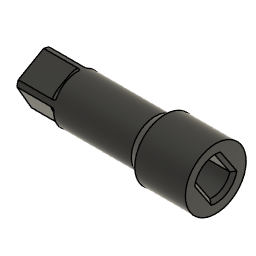
327ee1e9-15fe-45b5-88e0-88bf1f6365e6 (Autodesk Fusion 360 design; units mm, degrees)
Autodesk Fusion 360 part; units mm, degrees
sketch "Esboço1" plane through (-18.5, 0, 0) normal (-1, 0, 0) x (0, 0.065186, -0.997873)
  circle A0 centre (-39.8924, -6.2763) radius 4.5
  line L0 (-38.1174, -4.275) -> (-38.1174, -8.2775)
  line L1 (-41.6674, -4.275) -> (-41.6674, -8.2775)
  arc A1 (-41.6674, -8.2775) -> (-38.1174, -8.2775) centre (-39.8924, -6.2763) ccw
  arc A2 (-38.1174, -4.275) -> (-41.6674, -4.275) centre (-39.8924, -6.2763) ccw
  line L2 (-38.1174, -6.2763) -> (-41.6674, -6.2763) construction
  dimension "d5" = 9
  dimension "d16" = 5.35
  dimension "d18" = 3.55
  constraint vertical L1
  constraint coincident L0.start A1
  constraint concentric A1 A2
  constraint concentric A0 A2
  constraint coincident L0 L2.start
  constraint coincident L1 L2.end
  constraint perpendicular L1 L2
  constraint midpoint A0.centre L2
  constraint perpendicular L0 L2
  measures "d5" diameter of A0
  measures "d16" diameter of A1
  measures "d18" distance of L0 L1
extrude "Extrusão1" add sketch "Esboço1" against normal blind 7.5 contours A0 | L0 L1 A1 A2
sketch "Esboço2" plane through (-18.5, 0, 0) normal (-1, 0, 0) x (0, -1, 0)
  circle A0 centre (-3.6625, 40.2167) radius 4.5
  circle A1 centre (-3.6625, 40.2167) radius 3.5
  dimension "d9" = 7
  constraint concentric A0 A1
  measures "d9" diameter of A1
extrude "Extrusão3" cut sketch "Esboço1" against normal blind 7.5 contours L0 L1 A1 A2
extrude "Extrusão2" add sketch "Esboço2" along normal blind 13 contours A1
chamfer "Chanfro1" distance 1 distance2 1.5 1 edges at (-18.5, 6.9256, 41.4824) measured on face at (-18.5, 4.1672, 36.091)
sketch "Esboço3" plane through (-31.5, 0, 0) normal (-1, 0, 0) x (0, -1, 0)
  circle A0 centre (-3.6625, 40.2167) radius 3.5
  line L0 (-0.9125, 42.9667) -> (-6.4125, 42.9667)
  line L1 (-6.4125, 42.9667) -> (-6.4125, 37.4667)
  line L2 (-6.4125, 37.4667) -> (-0.9125, 37.4667)
  line L3 (-0.9125, 37.4667) -> (-0.9125, 42.9667)
  line L4 (-0.9125, 42.9667) -> (-6.4125, 37.4667) construction
  line L5 (-6.4125, 42.9667) -> (-0.9125, 37.4667) construction
  circle A1 centre (-3.6625, 40.2167) radius 1
  point P0 (-3.6625, 40.2167)
  dimension "d14" = 5.5
  dimension "d15" = 5.5
  dimension "d158" = 2
  constraint horizontal L0
  constraint perpendicular L0 L1
  constraint parallel L0 L2
  constraint parallel L1 L3
  constraint coincident L4 P0
  constraint coincident L5 P0
  constraint coincident P0 A0.centre
  measures "d14" distance of L1.end L2.end
  measures "d15" distance of L0.end L1.end
  measures "d158" diameter of A1
extrude "Extrusão4" add sketch "Esboço3" along normal blind 5.5 contours A0 L0 L1 L2 L3 | A1
fillet "Arredondamento1" radius 0.75 4 edges at (-31.5, 3.6625, 42.9667) (-31.5, 6.4125, 40.2167) (-31.5, 3.6625, 37.4667) (-31.5, 0.9125, 40.2167)
chamfer "Chanfro2" distance 0.5 angle 45 4 edges at (-11, 0.9932, 40.0424) (-11, 3.7782, 38.4455) (-11, 3.5468, 41.988) (-11, 6.3318, 40.3911)
extrude "Extrusão5" cut sketch "Esboço3" along normal blind 5.5 and the other way blind 4 contours A1
move_body "Mover1" bodies 1 to x (1, 0, 0) y (0, 0.5, -0.866025) z (0, 0.866025, 0.5) at (0, -32.9975, 23.2802)
